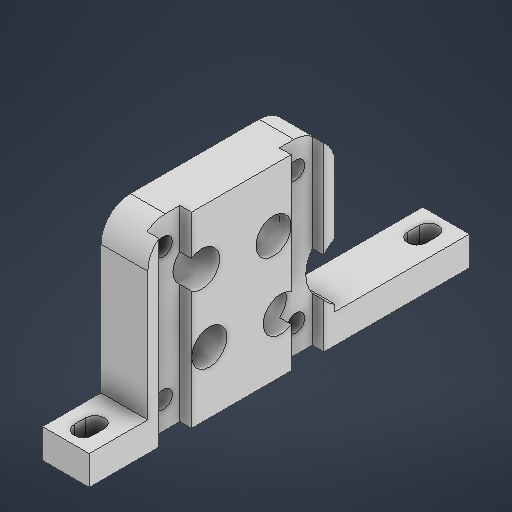
# Autodesk Inventor part: support_moteur_brushless2
Saved by Autodesk Inventor 2026.1 (Build 301233000, 233)
## iProperties
Created: 2022-10-25
Part Number: support_moteur_brushless2
Material: Générique
Document SubType Name: Modeling
Designer: ropertth
Density: 1 g/cm^3
Appearance: Par défaut
Mass: 7.3531 g
Surface Area: 46.1676 cm^2
Volume: 7.3531 cm^3
Author: ropertth
Autodesk Inventor part; units mm, degrees
ref_plane "YZ Plane" through (0, 0, 0) normal (1, 0, 0) x (0, 1, 0)
ref_plane "XZ Plane" through (0, 0, 0) normal (0, 1, 0) x (-1, 0, 0)
ref_plane "XY Plane" through (0, 0, 0) normal (0, 0, 1) x (1, 0, 0)
sketch "Esquisse1" plane through (0, 0, 0) normal (1, 0, 0) x (0, 1, 0)
  line L0 (0, 0) -> (5, 0)
  line L1 (5, 0) -> (5, -10)
  line L2 (5, -10) -> (32, -10)
  line L3 (32, -10) -> (32, -42)
  line L4 (32, -42) -> (5, -42)
  line L5 (5, -42) -> (5, -65)
  line L6 (5, -65) -> (0, -65)
  line L7 (0, -65) -> (0, 0)
  dimension "d0" = 5
  dimension "d1" = 32
  dimension "d2" = 32
  dimension "d3" = 10
  dimension "d4" = 65
  constraints: 16 end point, 6 perpendicular, 2 point on line, 1 horizontal
  measures "d0" distance between parallel lines of L1 L7
  measures "d1" distance between parallel lines of L3 L7
  measures "d2" distance of L2.end L3.end
  measures "d3" distance of L0.end L1.end
  measures "d4" distance of L6.end L0.start
extrude "Extrusion1" add sketch "Esquisse1" along normal blind 8
sketch "Esquisse2" plane through (8, 0, 0) normal (1, 0, 0) x (0, 0, -1)
  circle A0 centre (26, 16) radius 9.5 construction
  line L0 (0, 0) -> (65, 0) projected
  line L1 (10, 32) -> (10, 5) projected
  line L2 (26, 16) -> (19.2825, 22.7175) construction
  circle A1 centre (26, 16) radius 7.75 construction
  line L3 (26, 16) -> (20.5199, 10.5199) construction
  circle A2 centre (19.2825, 22.7175) radius 3
  circle A3 centre (20.5199, 10.5199) radius 3
  circle A4 centre (31.4801, 21.4801) radius 3
  circle A5 centre (32.7175, 9.2825) radius 3
  dimension "d9" = 19
  dimension "d7" = 16
  dimension "d8" = 16
  dimension "d10" = 45
  dimension "d11" = 15.5
  dimension "d12" = 45
  dimension "d13" = 6
  dimension "d14" = 6
  dimension "d31" = 360
  dimension "d35" = 360
  constraints: 5 centre point, 4 end point, 2 coincident, 2 point on circle, 13 other
  measures "d7" distance from line of L0 L2.start
  measures "d8" distance from line of L1 L2.start
  measures "d10" angle of L1 L2
  measures "d11" diameter of A1
  measures "d12" angle of L1 L3
  measures "d13" diameter of A2
  measures "d14" diameter of A3
extrude "Extrusion2" cut sketch "Esquisse2" against normal through all
sketch "Esquisse3" plane through (8, 0, 0) normal (1, 0, 0) x (0, 0, -1)
  circle A0 centre (26, 16) radius 16 construction
  line L0 (10, 32) -> (10, 5) projected
  line L1 (0, 0) -> (65, 0) projected
  line L2 (26, 16) -> (14.6863, 27.3137) construction
  line L3 (42, 32) -> (10, 32) projected
  circle A1 centre (14.6863, 27.3137) radius 1.5
  circle A2 centre (14.6863, 4.6863) radius 1.5
  circle A3 centre (37.3137, 4.6863) radius 1.5
  circle A4 centre (37.3137, 27.3137) radius 1.5
  dimension "d17" = 32
  dimension "d18" = 16
  dimension "d19" = 16
  dimension "d20" = 45
  dimension "d21" = 3
  dimension "d24" = 360
  constraints: 4 centre point, 2 end point, 1 coincident, 12 other
  measures "d18" distance from line of L0 L2.start
  measures "d19" distance from line of L1 L2.start
  measures "d20" angle of L3 L2
  measures "d21" diameter of A1
extrude "Extrusion3" cut sketch "Esquisse3" against normal through all
fillet "Congé1" radius 5 2 edges at (4, 32, -10) (4, 32, -42)
sketch "Esquisse4" plane through (0, 5, 0) normal (0, 1, 0) x (1, 0, 0)
  line L0 (4, 5) -> (4, 3) construction
  line L1 (2.4, 5) -> (2.4, 3)
  line L2 (5.6, 3) -> (5.6, 5)
  arc A0 (5.6, 5) -> (2.4, 5) centre (4, 5) ccw
  arc A1 (2.4, 3) -> (5.6, 3) centre (4, 3) ccw
  line L3 (0, 0) -> (8, 0) projected
  line L4 (0, 10) -> (0, 0) projected
  point P0 (4, 4)
  dimension "d37" = 3
  dimension "d38" = 2
  dimension "d39" = 4
  dimension "d40" = 1.6
  constraints: 8 end point, 4 point on circle, 4 tangent, 2 centre point, 1 midpoint, 1 parallel, 1 vertical
  measures "d37" distance from line of L3 L0.end
  measures "d38" distance of L0.start L0.end
  measures "d39" distance between parallel lines of L4 L0
  measures "d40" radius of A1
extrude "Extrusion4" cut sketch "Esquisse4" against normal through all
pattern_linear "Réseau rectangulaire1" count 2 spacing 57 along (0, 0, -1) of "Extrusion4"
sketch "Esquisse5" plane through (8, 0, 0) normal (1, 0, 0) x (0, 0, -1)
  line L0 (11.8863, 37.0839) -> (17.4863, 37.0839)
  line L1 (17.4863, 37.0839) -> (17.4863, -4.5812)
  line L2 (17.4863, -4.5812) -> (11.8863, -4.5812)
  line L3 (11.8863, -4.5812) -> (11.8863, 37.0839)
  circle A0 centre (14.6863, 27.3137) radius 1.5 projected
  line L4 (34.5137, 38.7224) -> (40.1137, 38.7224)
  line L5 (40.1137, 38.7224) -> (40.1137, -5.31)
  line L6 (40.1137, -5.31) -> (34.5137, -5.31)
  line L7 (34.5137, -5.31) -> (34.5137, 38.7224)
  circle A1 centre (37.3137, 27.3137) radius 1.5 projected
  point P0 (0, 0)
  dimension "d47" = 2.8
  dimension "d48" = 5.6
  dimension "d49" = 2.8
  dimension "d50" = 5.6
  constraints: 16 end point, 4 parallel, 2 horizontal, 2 perpendicular
  measures "d47" distance from line of A0.centre L3
  measures "d48" distance of L0.start L0.end
  measures "d49" distance from line of A1.centre L7
  measures "d50" distance of L4.start L4.end
extrude "Extrusion5" cut sketch "Esquisse5" against normal blind 2 contours L0 L1 L2 L3 | L4 L5 L6 L7 | A1
sketch "Esquisse6" plane through (8, 0, 0) normal (1, 0, 0) x (0, 0, -1)
  circle A0 centre (44.5, 11) radius 5.5
  line L0 (10, 27) -> (10, 5) projected
  line L1 (40.1137, 0) -> (11.8863, 0) projected
  point P0 (0, 0)
  point P1 (10, 7)
  point P2 (63, 0)
  dimension "d53" = 34.5
  dimension "d54" = 11
  dimension "d55" = 11
  constraints: 1 centre point
  measures "d53" distance from line of L0 A0.centre
  measures "d54" diameter of A0
  measures "d55" distance from line of L1 A0.centre
extrude "Extrusion6" cut sketch "Esquisse6" against normal through all
